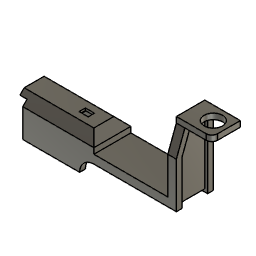
gas-meter-sensor-mount (Autodesk Fusion 360 design; units mm, degrees)
Autodesk Fusion 360 part; units mm, degrees
note: some values were not read from the file. Chosen so that the rebuilt part matches the saved one: which sketch regions a step uses; which pieces of a blend or face edit are solid.
sketch "Rahmen" plane through (0, 0, 0) normal (0, 1, 0) x (1, 0, 0) in component "Gehäuse"
  line L0 (0, 0) -> (0, -23)
  line L1 (0, -23) -> (12.5, -23)
  line L2 (12.5, -23) -> (12.5, -21)
  line L3 (12.5, -21) -> (3, -21)
  line L4 (3, -21) -> (3, 3)
  line L5 (3, 3) -> (-26, 3)
  line L6 (-51, -3.5) -> (-53.5, -3.5)
  line L7 (-53.5, -3.5) -> (-53.5, -5)
  line L8 (-53.5, -5) -> (-26, -5)
  line L9 (-26, -5) -> (-26, 0)
  line L10 (-26, 0) -> (0, 0)
  arc A0 (-31, 8) -> (-26, 3) centre (-26, 8) ccw
  line L11 (-51, 8) -> (-31, 8)
  line L12 (-51, -3.5) -> (-51, 8)
  dimension "d2" = 23
  dimension "d3" = 12.5
  dimension "d4" = 2
  dimension "d5" = 1.5
  dimension "d7" = 3
  dimension "d8" = 3
  dimension "d10" = 5
  dimension "d38" = 2.5
  dimension "d39" = 25
  dimension "d55" = 5
  dimension "d56" = 20
  dimension "d57" = 51
  dimension "d58" = 11.5
  dimension "d59" = 5
  constraint coincident L0.start L10.end
  constraint vertical L0
  constraint perpendicular L0 L1
  constraint perpendicular L1 L2
  constraint perpendicular L2 L3
  constraint perpendicular L3 L4
  constraint perpendicular L4 L5
  constraint perpendicular L6 L7
  constraint perpendicular L7 L8
  constraint perpendicular L8 L9
  constraint perpendicular L0 L10
  constraint perpendicular L11 L12
  constraint horizontal L8
  constraint vertical L12
  measures "d2" distance of L0.start L0.end
  measures "d3" distance of L0.end L1.end
  measures "d4" distance of L1.end L2.end
  measures "d5" distance of L6.end L7.end
  measures "d7" horizontal distance of L0.end L3.end
  measures "d8" vertical distance of L0.start L4.end
  measures "d10" distance of L8.end L9.end
  measures "d38" distance of L6.start L6.end
  measures "d39" horizontal distance of L6.start L8.end
  measures "d55" radius of A0
  measures "d56" distance of L11.start A0.start
  measures "d57" horizontal distance of L0.start L6.start
  measures "d58" distance of L6.start L11.start
  measures "d59" horizontal distance of L5.end A0.start
extrude "Extrude1" add sketch "Rahmen" against normal blind 13 makes body 1 in component "Gehäuse"
sketch "Loch" plane through (0, 0, 23) normal (0, 0, 1) x (-1, 0, 0) in component "Gehäuse"
  line L0 (-12.5, 0) -> (0, 0)
  line L1 (0, 0) -> (0, 13)
  line L2 (0, 13) -> (-12.5, 13)
  line L3 (-12.5, 13) -> (-12.5, 0)
  circle A0 centre (-7.75, 4.75) radius 3.25
  line L4 (0, 10) -> (-12.5, 10)
  line L5 (-12.5, 10) -> (-12.5, 13)
  line L6 (-12.5, 13) -> (0, 13)
  line L7 (0, 13) -> (0, 10)
  dimension "d13" = 7.75
  dimension "d14" = 4.75
  dimension "d15" = 6.5
  dimension "d16" = 3
  constraint horizontal L4
  constraint vertical L5
  constraint horizontal L6
  constraint vertical L7
  constraint coincident L2.end L3.start
  constraint coincident L1 L4.start
  measures "d13" horizontal distance of L0.end A0.centre
  measures "d14" vertical distance of L0.end A0.centre
  measures "d15" diameter of A0
  measures "d16" distance of L4.end L2.end
extrude "Extrude2" cut sketch "Loch" against normal blind 2 contours L1 L2 L3 L4 L5 L6 L7 | A0 bodies 1 in component "Gehäuse"
sketch "Sketch3" plane through (3, 0, 0) normal (1, 0, 0) x (0, 1, 0) in component "Gehäuse"
  line L0 (0, -3) -> (0, 21)
  line L1 (0, 21) -> (-10, 21)
  line L2 (-10, 21) -> (-13, 21)
  line L3 (-13, 21) -> (-13, -3)
  line L4 (-13, -3) -> (0, -3)
  line L5 (-10, 21) -> (-10, 13)
  line L6 (-10, 21) -> (-13, 13)
  line L7 (-13, 13) -> (-10, 13)
  dimension "d19" = 8
  constraint coincident L1.end L2.start
  constraint perpendicular L1 L5
  constraint coincident L3 L6.end
  constraint perpendicular L5 L7
  measures "d19" vertical distance of L1.end L6.end
extrude "Extrude3" cut sketch "Sketch3" against normal blind 3 contours L2 L3 L6 bodies 1 in component "Gehäuse"
fillet "Fillet1" radius 2 1 edges at (12.5, -10, 22) on bodies 1 in component "Gehäuse"
chamfer "Chamfer1" distance 3 angle 45 3 edges at (-26, -6.5, 5) (-39.75, 0, 5) (-39.75, -13, 5) on bodies 1 in component "Gehäuse"
shell "Shell3" thickness 2 removed faces 4 at (3, -4.3333, 10.3333) at (-6.6667, -8.6667, -3) at (-27.6353, -8.6667, -3.275) at (-44.3333, -8.6667, -8) on bodies 1 in component "Gehäuse"
sketch "Sensor" plane through (0, 0, 3) normal (0, 0, -1) x (1, 0, 0) in component "Gehäuse"
  line L0 (-49, 3.8284) -> (-29.8284, 3.8284)
  line L1 (-29.8284, 3.8284) -> (-29.8284, 9.1716)
  line L2 (-29.8284, 9.1716) -> (-49, 9.1716)
  line L3 (-37.6, 9.1) -> (-32.4, 9.1)
  line L4 (-32.4, 9.1) -> (-32.4, 3.9)
  line L5 (-32.4, 3.9) -> (-37.6, 3.9)
  line L6 (-37.6, 3.9) -> (-37.6, 9.1)
  line L7 (-49, 6.5) -> (-11.5826, 6.5) construction
  line L8 (-49, 9.1716) -> (-49, 3.8284)
  line L9 (-36.6, 5.4) -> (-33.4, 5.4)
  line L10 (-33.4, 5.4) -> (-33.4, 7.6)
  line L11 (-33.4, 7.6) -> (-36.6, 7.6)
  line L12 (-36.6, 7.6) -> (-36.6, 5.4)
  line L13 (-35, -1.9581) -> (-35, 14.9581) construction
  dimension "d43" = 5.2
  dimension "d45" = 5.2
  dimension "d111" = 3.2
  dimension "d112" = 2.2
  dimension "d114" = 35
  constraint perpendicular L1 L7
  constraint symmetric L3 L5 L7
  constraint midpoint L7.start L8
  constraint symmetric L7 L9 L11
  constraint symmetric L7 L13.start L13.end
  constraint symmetric L4 L6 L13
  constraint vertical L4
  constraint horizontal L3
  constraint vertical L10
  constraint horizontal L11
  measures "d43" distance of L3.start L3.end
  measures "d45" distance of L3.end L4.end
  measures "d111" distance of L9.start L9.end
  measures "d112" distance of L9.start L11.end
  measures "d114" horizontal distance of origin L13.start
extrude "Extrude6" cut sketch "Sensor" against normal blind 1.2 contours L3 L4 L5 L6 | L9 L10 L11 L12 bodies 1 in component "Gehäuse"
extrude "Extrude7" cut sketch "Sensor" against normal up to surface (2 mm away) contours L9 L10 L11 L12 bodies 1 in component "Gehäuse"
hole "Hole1" at (-51, -6.5, -5) direction (1, 0, 0) diameter 4.2 depth 2 tip angle 180 bodies 1 in component "Gehäuse"
sketch "Clip" plane through (0, 0, 0) normal (0, 1, 0) x (1, 0, 0) in component "Clip"
  line L0 (-4.5, -1) -> (-3, -1)
  line L1 (-3, -1) -> (-3, -8)
  line L2 (-3, -8) -> (-3.5, -8)
  line L3 (-3.5, -8) -> (-3, -9.5)
  line L4 (-3, -9.5) -> (0, -9.5)
  line L5 (0, -9.5) -> (0, 0)
  line L6 (-0.5, -9.5) -> (0.5, -9.5)
  line L7 (0.5, -9.5) -> (0.5, -2.5)
  line L8 (-0.5, -2.5) -> (-0.5, -9.5)
  line L9 (-0.5, -9.5) -> (0.5, -2) construction
  line L10 (-0.5, -2) -> (0.5, -9.5) construction
  line L11 (-4.5, -1) -> (-4.5, 0)
  line L12 (0, 0) -> (-4.5, 0)
  line L13 (0, -2) -> (-0.0001, -2)
  arc A0 (0, -2) -> (-0.5, -2.5) centre (0, -2.5) ccw
  arc A1 (0.5, -2.5) -> (-0.0001, -2) centre (0, -2.5) ccw
  point P0 (0, -5.75)
  dimension "d79" = 0.5
  dimension "d81" = 3
  dimension "d84" = 1
  dimension "d90" = 1.5
  dimension "d91" = 3
  dimension "d92" = 7
  dimension "d97" = 4.5
  dimension "d98" = 1
  dimension "d107" = 2
  dimension "d108" = 0.5
  constraint perpendicular L0 L1
  constraint perpendicular L1 L2
  constraint coincident L5.end L12.start
  constraint horizontal L6
  constraint vertical L7
  constraint vertical L8
  constraint coincident L4 L6.start
  constraint midpoint L9 P0
  constraint coincident L5 P0
  constraint horizontal L4
  constraint vertical L1
  constraint horizontal L12
  constraint vertical L11
  constraint vertical L5
  constraint coincident L10.start L8
  constraint coincident L9.end L7
  constraint horizontal L13
  constraint coincident L10.start L13
  constraint tangent L8 A0
  constraint tangent L13 A0
  constraint coincident L9.end L13
  constraint equal A0 A1
  constraint tangent L7 A1
  constraint tangent A0 A1
  measures "d79" distance of L1.end L2.end
  measures "d81" horizontal distance of L5.end L0.end
  measures "d84" distance of L6.start L6.end
  measures "d90" vertical distance of L1.end L3.end
  measures "d91" horizontal distance of L3.end L4.end
  measures "d92" distance of L0.end L1.end
  measures "d97" horizontal distance of L11.end L5.end
  measures "d98" vertical distance of L0.start L11.end
  measures "d107" distance of L5.end L13
  measures "d108" radius of A0
revolve "Revolve1" add sketch "Clip" angle 360 about axis through (0, 0, 9.5) along (0, 0, -1) separate body contours L0 L1 L2 L3 L4 L5 L8 L11 L12 A0 | L4 L5 L6 L8 A0 makes body 2 in component "Clip"
extrude "Extrude4" cut sketch "Clip" along normal through all and the other way through all contours L5 L6 L7 A1 | L4 L5 L6 L8 A0 bodies 2 in component "Clip"
fillet "Fillet1'" radius 0.5 1 edges at (-2.797, 1.0848, 1) on bodies 2 in component "Clip"
fillet "Fillet2" radius 0.25 1 edges at (-4.1955, 1.6273, 0) on bodies 2 in component "Clip"
component "Gehäuse" placed x (1, 0, 0) y (0, 1, 0) z (0, 0, 1) at (0, 0, 0)
component "Clip" placed x (1, 0, 0) y (0, 1, 0) z (0, 0, 1) at (7.75, -4.75, 19)
named bodies: "Body", "Bolzen"
